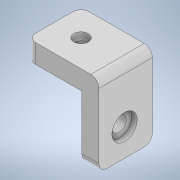
# Autodesk Inventor part: soportetuerca
Saved by Autodesk Inventor 2022 (Build 260153000, 153)
## iProperties
Created: 2022-03-05
Part Number: soportetuerca
Material: Genérico
Document SubType Name: Modeling
Designer: JK
Density: 1 g/cm^3
Appearance: Valor por defecto
Author: JK
Autodesk Inventor part; units mm, degrees
ref_plane "YZ Plane" through (0, 0, 0) normal (1, 0, 0) x (0, 1, 0)
ref_plane "XZ Plane" through (0, 0, 0) normal (0, 1, 0) x (-1, 0, 0)
ref_plane "XY Plane" through (0, 0, 0) normal (0, 0, 1) x (1, 0, 0)
sketch "Boceto1" plane through (0, 0, 0) normal (0, 1, 0) x (-1, 0, 0)
  line L0 (-9.85, 9.85) -> (9.85, 9.85)
  line L1 (9.85, 9.85) -> (9.85, -9.85)
  line L2 (9.85, -9.85) -> (-9.85, -9.85)
  line L3 (-9.85, -9.85) -> (-9.85, 9.85)
  line L4 (-9.85, 9.85) -> (9.85, -9.85) construction
  line L5 (9.85, 9.85) -> (-9.85, -9.85) construction
  point P0 (0, 0)
  dimension "d0" = 19.7
  dimension "d1" = 19.7
  constraints: 12 end point, 2 midpoint, 2 parallel, 1 horizontal, 1 perpendicular
  measures "d0" distance of L1.end L2.end
  measures "d1" distance of L0.end L1.end
extrude "Extrusión1" add sketch "Boceto1" along normal blind 7
sketch "Boceto2" plane through (0, 7, 0) normal (0, 1, 0) x (1, 0, 0)
  line L0 (-9.85, -9.85) -> (9.85, -9.85) projected
  line L1 (9.85, -9.85) -> (16.45, -9.85)
  line L2 (16.45, -9.85) -> (16.45, 9.85)
  line L3 (16.45, 9.85) -> (9.85, 9.85)
  line L4 (9.85, 9.85) -> (9.85, -9.85)
  line L5 (9.85, 9.85) -> (-9.85, 9.85) projected
  point P0 (0, 0)
  dimension "d4" = 6.6
  constraints: 8 end point, 2 parallel, 1 collinear, 1 horizontal, 1 perpendicular
  measures "d4" distance between parallel lines of L4 L2
extrude "Extrusión2" add sketch "Boceto2" against normal blind 30
sketch "Boceto3" plane through (16.45, 7, 9.85) normal (1, 0, 0) x (0, 0, -1)
  circle A0 centre (9.435, -20) radius 2.7
  line L0 (19.7, -30) -> (0, -30) projected
  point P0 (9.85, -7)
  dimension "d7" = 5.4
  dimension "d8" = 10
  constraints: 1 centre point
  measures "d7" diameter of A0
  measures "d8" distance from line of A0.centre L0
extrude "Extrusión3" cut sketch "Boceto3" against normal blind 20
sketch "Boceto4" plane through (16.45, 7, 9.85) normal (1, 0, 0) x (0, 0, -1)
  circle A0 centre (9.435, -20) radius 2.7 projected
  circle A1 centre (9.435, -20) radius 4.65
  point P0 (9.85, -7)
  dimension "d11" = 9.3
  constraints: 1 centre point, 1 coincident
  measures "d11" diameter of A1
extrude "Extrusión4" cut sketch "Boceto4" against normal blind 2 contours A0 | A1
sketch "Boceto5" plane through (0, 7, 0) normal (0, 1, 0) x (1, 0, 0)
  circle A0 centre (0, 0) radius 2.7
  dimension "d14" = 5.4
  constraints: 1 centre point, 1 coincident
  measures "d14" diameter of A0
extrude "Extrusión5" cut sketch "Boceto5" against normal through all
sketch "Boceto6" plane through (0, 0, 0) normal (0, -1, 0) x (1, 0, 0)
  circle A0 centre (0, 0) radius 4.05
  line L0 (0, 4.6765) -> (4.05, 2.3383)
  line L1 (4.05, 2.3383) -> (4.05, -2.3383)
  line L2 (4.05, -2.3383) -> (0, -4.6765)
  line L3 (0, -4.6765) -> (-4.05, -2.3383)
  line L4 (-4.05, -2.3383) -> (-4.05, 2.3383)
  line L5 (-4.05, 2.3383) -> (0, 4.6765)
  dimension "d17" = 8.1
  constraints: 12 end point, 2 coincident, 1 centre point, 1 tangent, 13 other
  measures "d17" diameter of A0
extrude "Extrusión6" cut sketch "Boceto6" against normal blind 4.1
fillet "Empalme1" radius 3 3 edges at (16.45, 7, 0) (13.15, -23, 9.85) (13.15, -23, -9.85)
sketch "Boceto8" plane through (0, 0, 0) normal (0, -1, 0) x (1, 0, 0)
  line L0 (10.15, -10.15) -> (-10.15, -10.15)
  line L1 (-10.15, -10.15) -> (-10.15, 10.15)
  line L2 (-10.15, 10.15) -> (10.15, 10.15)
  line L3 (10.15, 10.15) -> (10.15, -10.15)
  line L4 (10.15, -10.15) -> (-10.15, 10.15) construction
  line L5 (-10.15, -10.15) -> (10.15, 10.15) construction
  point P0 (0, 0)
  dimension "d21" = 20.3
  dimension "d22" = 20.3
  constraints: 12 end point, 2 midpoint, 2 parallel, 1 horizontal, 1 perpendicular
  measures "d21" distance of L1.end L2.end
  measures "d22" distance of L0.end L1.end
extrude "Extrusión7" cut sketch "Boceto8" along normal through all
fillet "Empalme2" radius 3 2 edges at (-9.85, 3.5, 9.85) (-9.85, 3.5, -9.85)
